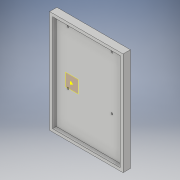
# Autodesk Inventor part: Robot_Base
Saved by Autodesk Inventor 2019.4 (Build 234330000, 330)
## iProperties
Created: 2019-09-20
Part Number: Robot_Base
Material: Generic
Document SubType Name: Modeling
Designer: Pranav Maddula
Density: 1 g/cm^3
Appearance: Default
Author: Pranav Maddula
Autodesk Inventor part; units mm, degrees
ref_plane "YZ Plane" through (0, 0, 0) normal (1, 0, 0) x (0, 1, 0)
ref_plane "XZ Plane" through (0, 0, 0) normal (0, 1, 0) x (-1, 0, 0)
ref_plane "XY Plane" through (0, 0, 0) normal (0, 0, 1) x (1, 0, 0)
sketch "Sketch1" plane through (0, 0, 0) normal (0, 0, 1) x (1, 0, 0)
  line L0 (-31.9998, 94.2737) -> (95.0002, 94.2737)
  line L1 (95.0002, 94.2737) -> (95.0002, -83.5263)
  line L2 (95.0002, -83.5263) -> (-31.9998, -83.5263)
  line L3 (-31.9998, -83.5263) -> (-31.9998, 94.2737)
  point P0 (0, 0)
  dimension "d0" = 127
  dimension "d1" = 177.8
  constraints: 8 end point, 2 parallel, 1 horizontal, 1 perpendicular
  measures "d0" distance of L0.start L0.end
  measures "d1" distance of L0.end L1.end
ref_plane "Work Plane1" through (0, 0, 6.35) normal (0, 0, 1) x (1, 0, 0)
sketch "Sketch3" plane through (0, 0, 6.35) normal (0, 0, 1) x (1, 0, 0)
  circle A0 centre (-6.5998, 81.5737) radius 1.7145
  line L0 (-57.3998, 94.2737) -> (-57.3998, -108.9263) projected
  circle A1 centre (69.6002, 81.5737) radius 1.7145
  circle A2 centre (-6.5998, -11.1363) radius 1.7145
  circle A3 centre (69.6002, -11.1363) radius 1.7145
  line L1 (95.0002, -108.9263) -> (95.0002, 94.2737) projected
  line L2 (95.0002, 94.2737) -> (-57.3998, 94.2737) projected
  point P0 (0, 0)
  dimension "d4" = 3.429
  dimension "d7" = 50.8
  dimension "d14" = 3.429
  dimension "d15" = 3.429
  dimension "d16" = 3.429
  dimension "d17" = 76.2
  dimension "d18" = 92.71
  dimension "d19" = 92.71
  dimension "d20" = 76.2
  dimension "d21" = 25.4
  dimension "d22" = 12.7
  dimension "d23" = 12.7
  constraints: 4 centre point
  measures "d4" diameter of A0
  measures "d7" distance from line of L0 A0.centre
  measures "d14" diameter of A1
  measures "d15" diameter of A2
  measures "d16" diameter of A3
  measures "d17" distance of A1.centre A0.centre
  measures "d18" distance of A2.centre A0.centre
  measures "d19" distance of A3.centre A1.centre
  measures "d20" distance of A3.centre A2.centre
  measures "d21" distance from line of L1 A3.centre
  measures "d22" distance from line of L2 A0.centre
  measures "d23" distance from line of L2 A1.centre
extrude "Extrusion3" add sketch "Sketch1" along normal blind 6.35
extrude "Extrusion4" cut sketch "Sketch3" against normal blind 6.35
sketch "Sketch4" plane through (0, 0, 6.35) normal (0, 0, 1) x (1, 0, 0)
  point P0 (0, 0)
sketch "Sketch6" plane through (0, 0, 6.35) normal (0, 0, 1) x (1, 0, 0)
  line L0 (-31.9998, 94.2737) -> (-31.9998, -83.5263) projected
  line L1 (-31.9998, 94.2737) -> (-26.9198, 94.2737)
  line L2 (-26.9198, 94.2737) -> (-26.9198, -83.5263)
  line L3 (-26.9198, -83.5263) -> (-31.9998, -83.5263)
  line L4 (-31.9998, -83.5263) -> (-31.9998, 94.2737)
  line L5 (95.0002, -83.5263) -> (95.0002, 94.2737) projected
  line L6 (-31.9998, -83.5263) -> (95.0002, -83.5263) projected
  line L7 (95.0002, 94.2737) -> (89.9202, 94.2737)
  line L8 (89.9202, 94.2737) -> (89.9202, -83.5263)
  line L9 (89.9202, -83.5263) -> (95.0002, -83.5263)
  line L10 (95.0002, -83.5263) -> (95.0002, 94.2737)
  line L11 (-26.9198, 94.2737) -> (89.9202, 94.2737)
  line L12 (89.9202, 94.2737) -> (89.9202, 89.1937)
  line L13 (89.9202, 89.1937) -> (-26.9198, 89.1937)
  line L14 (-26.9198, 89.1937) -> (-26.9198, 94.2737)
  line L15 (-26.9198, -83.5263) -> (89.9202, -83.5263)
  line L16 (89.9202, -83.5263) -> (89.9202, -78.4463)
  line L17 (89.9202, -78.4463) -> (-26.9198, -78.4463)
  line L18 (-26.9198, -78.4463) -> (-26.9198, -83.5263)
  point P0 (0, 0)
  dimension "d34" = 5.08
  dimension "d35" = 5.08
  dimension "d36" = 5.08
  dimension "d37" = 5.08
  constraints: 32 end point, 8 parallel, 4 horizontal, 4 perpendicular, 3 point on line
  measures "d34" distance of L2.end L3.end
  measures "d35" distance of L9.end L8.end
  measures "d36" distance of L11.end L12.end
  measures "d37" distance of L16.end L15.end
extrude "Extrusion5" add sketch "Sketch6" along normal blind 6.35 contours L1 L2 L3 L0
sketch "Sketch7" plane through (0, 0, 6.35) normal (0, 0, 1) x (1, 0, 0)
  line L0 (-26.9198, 94.2737) -> (-31.9998, 94.2737) projected
  line L1 (95.0002, -83.5263) -> (95.0002, 94.2737) projected
  line L2 (-26.9198, 94.2737) -> (95.0002, 94.2737)
  line L3 (95.0002, 94.2737) -> (95.0002, 89.1937)
  line L4 (95.0002, 89.1937) -> (-26.9198, 89.1937)
  line L5 (-26.9198, 89.1937) -> (-26.9198, 94.2737)
  point P0 (0, 0)
  dimension "d40" = 5.08
  constraints: 8 end point, 2 parallel, 1 horizontal, 1 perpendicular, 1 point on line
  measures "d40" distance of L2.end L3.end
extrude "Extrusion6" add sketch "Sketch7" along normal blind 6.35
sketch "Sketch8" plane through (0, 0, 6.35) normal (0, 0, 1) x (1, 0, 0)
  line L0 (95.0002, 89.1937) -> (95.0002, 94.2737) projected
  line L1 (95.0002, 89.1937) -> (89.9202, 89.1937)
  line L2 (89.9202, 89.1937) -> (89.9202, -83.5263)
  line L3 (89.9202, -83.5263) -> (95.0002, -83.5263)
  line L4 (95.0002, -83.5263) -> (95.0002, 89.1937)
  point P0 (0, 0)
  dimension "d43" = 5.08
  dimension "d44" = 172.72
  constraints: 8 end point, 2 parallel, 1 horizontal, 1 perpendicular
  measures "d43" distance of L3.end L2.end
  measures "d44" distance of L2.end L1.end
extrude "Extrusion7" add sketch "Sketch8" along normal blind 6.35
sketch "Sketch9" plane through (0, 0, 6.35) normal (0, 0, 1) x (1, 0, 0)
  line L0 (89.9202, 89.1937) -> (89.9202, -83.5263) projected
  line L1 (89.9202, -83.5263) -> (-26.9198, -83.5263)
  line L2 (-26.9198, -83.5263) -> (-26.9198, -78.4463)
  line L3 (-26.9198, -78.4463) -> (89.9202, -78.4463)
  line L4 (89.9202, -78.4463) -> (89.9202, -83.5263)
  point P0 (0, 0)
  dimension "d47" = 116.84
  dimension "d48" = 5.08
  constraints: 8 end point, 2 parallel, 1 horizontal, 1 perpendicular
  measures "d47" distance of L2.end L3.end
  measures "d48" distance of L1.end L2.end
extrude "Extrusion8" add sketch "Sketch9" along normal blind 6.35
body "Solid1"
